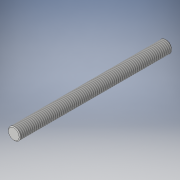
# Autodesk Inventor part: Направляющая
Saved by Autodesk Inventor 2017 (Build 210142000, 142)
## iProperties
Part Number: Направляющая
Material: Типовые
Document SubType Name: Modeling
Designer: Daemon
Density: 1 g/cm^3
Appearance: По умолчанию
Author: Daemon
Autodesk Inventor part; units mm, degrees
ref_plane "YZ Plane" through (0, 0, 0) normal (1, 0, 0) x (0, 1, 0)
ref_plane "XZ Plane" through (0, 0, 0) normal (0, 1, 0) x (-1, 0, 0)
ref_plane "XY Plane" through (0, 0, 0) normal (0, 0, 1) x (1, 0, 0)
sketch "Эскиз1" plane through (0, 0, 0) normal (0, 0, 1) x (1, 0, 0)
  circle A0 centre (0, 0) radius 4
  dimension "d0" = 8
  constraints: 1 centre point, 1 coincident
  measures "d0" diameter of A0
extrude "Выдавливание1" add sketch "Эскиз1" along normal blind 100
thread "Резьба1" size "M8x1.25" class "6g" standard "ANSI Metric M Profile" full length
chamfer "Фаска1" distance 0.5 angle 45 1 edges at (-4, 0, 100)
chamfer "Фаска2" distance 0.5 angle 45 1 edges at (-4, 0, 0)
